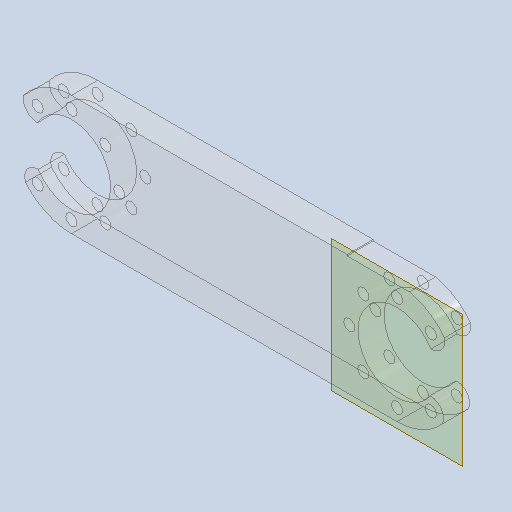
# Autodesk Inventor part: 0904_joint
Saved by Autodesk Inventor 2024.3 (Build 283343000, 343)
## iProperties
Created: 2024-09-04
Part Number: 0904_joint
Material: PMMA 플라스틱
Document SubType Name: Modeling
Designer: gretc
Density: 1.188 g/cm^3
Appearance: 폴리카보네이트 - 선명
Author: gretc
Autodesk Inventor part; units mm, degrees
ref_plane "YZ Plane" through (0, 0, 0) normal (1, 0, 0) x (0, 1, 0)
ref_plane "XZ Plane" through (0, 0, 0) normal (0, 1, 0) x (-1, 0, 0)
ref_plane "XY Plane" through (0, 0, 0) normal (0, 0, 1) x (1, 0, 0)
ref_plane "작업 평면1" through (0, 0, -52) normal (0, 0, -1) x (0, -1, 0)
sketch "스케치1" plane through (0, 0, -52) normal (0, 0, -1) x (0, -1, 0)
  circle A0 centre (0, 0) radius 13.8 projected
  circle A1 centre (0, 0) radius 7.2 projected
  circle A2 centre (0, -11) radius 1.2812 projected
  circle A3 centre (-7.7782, -7.7782) radius 1.2812 projected
  circle A4 centre (-11, 0) radius 1.2812 projected
  circle A5 centre (-7.7782, 7.7782) radius 1.2812 projected
  circle A6 centre (0, 11) radius 1.2812 projected
  circle A7 centre (7.7782, 7.7782) radius 1.2812 projected
  circle A8 centre (11, 0) radius 1.2812 projected
  circle A9 centre (7.7782, -7.7782) radius 1.2812 projected
  circle A10 centre (0, 0) radius 9 projected
  line L0 (-13.8, 0) -> (-13.8, 75.06)
  line L1 (13.8, 0) -> (13.8, 75.9397)
  line L2 (-13.5, -42) -> (-13.5, 11.5) projected
  line L3 (-13.5, -42) -> (-14.5, -42) projected
  line L4 (-14.5, -42) -> (-14.5, 11.5) projected
  line L5 (-13.5, 11.5) -> (-14.5, 11.5) projected
  circle A11 centre (0, 75) radius 13.8 projected
  circle A12 centre (0, 75) radius 7.2 projected
  circle A13 centre (0, 64) radius 1.2812 projected
  circle A14 centre (-7.7782, 67.2218) radius 1.2812 projected
  circle A15 centre (-11, 75) radius 1.2812 projected
  circle A16 centre (-7.7782, 82.7782) radius 1.2812 projected
  circle A17 centre (0, 86) radius 1.2812 projected
  circle A18 centre (7.7782, 82.7782) radius 1.2812 projected
  circle A19 centre (11, 75) radius 1.2812 projected
  circle A20 centre (7.7782, 67.2218) radius 1.2812 projected
  circle A21 centre (0, 75) radius 9 projected
  circle A22 centre (0, 75) radius 7.2 projected
  circle A23 centre (-7.7782, -7.7782) radius 3.2245
  circle A24 centre (7.7782, -7.7782) radius 2.9483
  circle A25 centre (7.7782, 82.7782) radius 3.0106
  circle A26 centre (-7.7782, 82.7782) radius 3.389
  point P0 (0, 0)
  point P1 (-4.5537, -7.763)
  point P2 (4.8359, -7.5904)
  point P3 (9, -10.4614)
  point P4 (13.8, 75.0006)
  point P5 (8.8434, 85.5941)
  point P6 (4.7711, 82.6313)
  point P7 (-4.3901, 82.8567)
  point P8 (-8.1333, 86.1485)
  point P9 (-13.8, 75)
  point P10 (-13.8, 11.5)
  point P11 (-13.5, -2.8618)
  point P12 (-8.412, -10.9398)
  dimension "d3" = 75.06
  dimension "d4" = 27.6
  dimension "d5" = 6.449
  dimension "d6" = 5.8966
  dimension "d7" = 6.778
  dimension "d8" = 6.0213
  constraints: 4 centre point, 4 coincident, 4 end point, 2 point on circle, 2 vertical, 1 tangent
  measures "d3" distance of L0.start L0.end
  measures "d4" distance between parallel lines of L1 L0
  measures "d5" diameter of A23
  measures "d6" diameter of A24
  measures "d7" diameter of A26
  measures "d8" diameter of A25
extrude "돌출1" add sketch "스케치1" along normal blind 6 contours A0 A24 A10 A23 L2 | A11 A26 A21 A25 | A0 L2 L5 L0 A11 L1 | A0 A24 A10 | A25 A21 A11 | A23 A10 A0 | A11 A26 A21 picked at (4.9363, 65.006)
